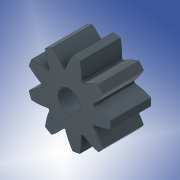
# Autodesk Inventor part: Motor Gear
Saved by Autodesk Inventor 2017 (Build 210142000, 142)
## iProperties
Created: 2017-07-05
Part Number: Motor Gear
Material: ABS Plastic
Document SubType Name: Modeling
Designer: zallen
Density: 1.06 g/cm^3
Appearance: CR Dark Blue
Author: zallen
Autodesk Inventor part; units mm, degrees
ref_plane "YZ Plane" through (0, 0, 0) normal (1, 0, 0) x (0, 1, 0)
ref_plane "XZ Plane" through (0, 0, 0) normal (0, 1, 0) x (-1, 0, 0)
ref_plane "XY Plane" through (0, 0, 0) normal (0, 0, 1) x (1, 0, 0)
sketch "Sketch1" plane through (0, 0, 0) normal (0, 0, 1) x (1, 0, 0)
  circle A0 centre (0, 0) radius 6.5
  line L0 (0, 0) -> (16, 0) construction
  arc A1 (10.1847, 0.9) -> (6.1847, 2) centre (4.2455, -12.8741) ccw
  arc A2 (6.1847, -2) -> (10.1847, -0.9) centre (4.2455, 12.8741) ccw
  arc A3 (6.1847, -2) -> (6.1847, 2) centre (0, 0) ccw
  arc A4 (10.1847, -0.9) -> (10.1847, 0.9) centre (-9.7951, 0) ccw
  arc A5 (7.2234, 7.236) -> (3.4521, 5.5075) centre (11.5276, -7.1332) ccw
  arc A6 (8.3804, 5.8571) -> (7.2234, 7.236) centre (-7.5035, -6.2962) ccw
  arc A7 (6.0233, 2.4433) -> (8.3804, 5.8571) centre (-5.0231, 12.5911) ccw
  arc A8 (6.0233, 2.4433) -> (3.4521, 5.5075) centre (0, 0) ccw
  arc A9 (0.8822, 10.1862) -> (-0.8957, 6.438) centre (13.4158, 1.9455) ccw
  arc A10 (2.6549, 9.8736) -> (0.8822, 10.1862) centre (-1.7009, -9.6463) ccw
  arc A11 (3.0436, 5.7434) -> (2.6549, 9.8736) centre (-11.9413, 6.4166) ccw
  arc A12 (3.0436, 5.7434) -> (-0.8957, 6.438) centre (0, 0) ccw
  arc A13 (-5.8718, 8.3702) -> (-4.8244, 4.3561) centre (9.0266, 10.1138) ccw
  arc A14 (-4.3129, 9.2702) -> (-5.8718, 8.3702) centre (4.8975, -8.4828) ccw
  arc A15 (-1.3603, 6.3561) -> (-4.3129, 9.2702) centre (-13.2721, -2.7603) ccw
  arc A16 (-1.3603, 6.3561) -> (-4.8244, 4.3561) centre (0, 0) ccw
  arc A17 (-9.8783, 2.6376) -> (-6.4957, 0.2359) centre (0.4137, 13.5498) ccw
  arc A18 (-9.2626, 4.3291) -> (-9.8783, 2.6376) centre (9.2044, -3.3501) ccw
  arc A19 (-5.1276, 3.9947) -> (-9.2626, 4.3291) centre (-8.3927, -10.6457) ccw
  arc A20 (-5.1276, 3.9947) -> (-6.4957, 0.2359) centre (0, 0) ccw
  arc A21 (-9.2626, -4.3291) -> (-5.1276, -3.9947) centre (-8.3927, 10.6457) ccw
  arc A22 (-9.8783, -2.6376) -> (-9.2626, -4.3291) centre (9.2044, 3.3501) ccw
  arc A23 (-6.4957, -0.2359) -> (-9.8783, -2.6376) centre (0.4137, -13.5498) ccw
  arc A24 (-6.4957, -0.2359) -> (-5.1276, -3.9947) centre (0, 0) ccw
  arc A25 (-4.3129, -9.2702) -> (-1.3603, -6.3561) centre (-13.2721, 2.7603) ccw
  arc A26 (-5.8718, -8.3702) -> (-4.3129, -9.2702) centre (4.8975, 8.4828) ccw
  arc A27 (-4.8244, -4.3561) -> (-5.8718, -8.3702) centre (9.0266, -10.1138) ccw
  arc A28 (-4.8244, -4.3561) -> (-1.3603, -6.3561) centre (0, 0) ccw
  arc A29 (2.6549, -9.8736) -> (3.0436, -5.7434) centre (-11.9413, -6.4166) ccw
  arc A30 (0.8822, -10.1862) -> (2.6549, -9.8736) centre (-1.7009, 9.6463) ccw
  arc A31 (-0.8957, -6.438) -> (0.8822, -10.1862) centre (13.4158, -1.9455) ccw
  arc A32 (-0.8957, -6.438) -> (3.0436, -5.7434) centre (0, 0) ccw
  arc A33 (8.3804, -5.8571) -> (6.0233, -2.4433) centre (-5.0231, -12.5911) ccw
  arc A34 (7.2234, -7.236) -> (8.3804, -5.8571) centre (-7.5035, 6.2962) ccw
  arc A35 (3.4521, -5.5075) -> (7.2234, -7.236) centre (11.5276, 7.1332) ccw
  arc A36 (3.4521, -5.5075) -> (6.0233, -2.4433) centre (0, 0) ccw
  point P0 (10.2049, 0)
  point P1 (7.8174, 6.5596)
  point P2 (1.7721, 10.0499)
  point P3 (-5.1025, 8.8377)
  point P4 (-9.5895, 3.4903)
  point P5 (-9.5895, -3.4903)
  point P6 (-5.1025, -8.8377)
  point P7 (1.7721, -10.0499)
  point P8 (7.8174, -6.5596)
  dimension "d0" = 13
  dimension "d1" = 16
  dimension "d2" = 15
  dimension "d3" = 4
  dimension "d4" = 2
  dimension "d6" = 1.8
  dimension "d15" = 20
  dimension "d18" = 360
  constraints: 73 point on circle, 36 centre point, 3 symmetric about line, 2 end point, 1 coincident, 1 horizontal, 1 point on line, 124 other
  measures "d1" distance of L0.start L0.end
  measures "d2" radius of A1
  measures "d3" horizontal distance of A1.start A1.end
  measures "d4" distance from line of L0 A1.end
  measures "d6" distance of A2.end A1.start
  measures "d15" radius of A4
extrude "Extrusion1" add sketch "Sketch1" along normal blind 10
sketch "Sketch5" plane through (0, 0, 10) normal (0, 0, 1) x (1, 0, 0)
  circle A0 centre (0, 0) radius 2.75
  dimension "d32" = 5.5
  constraints: 1 centre point, 1 coincident
  measures "d32" diameter of A0
extrude "Extrusion5" cut sketch "Sketch5" against normal through all
body "Solid1"
